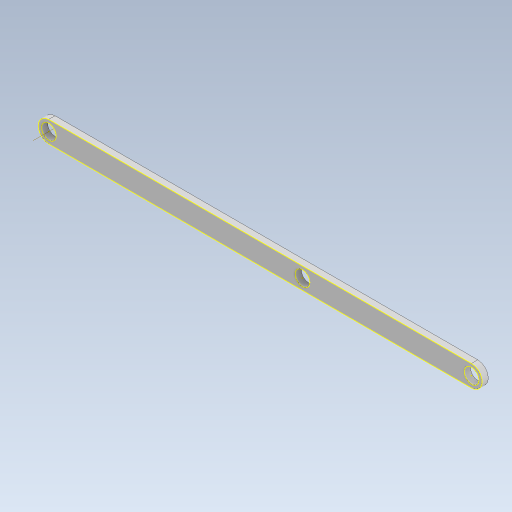
# Autodesk Inventor part: 0605_2
Saved by Autodesk Inventor 2023 (Build 270158000, 158)
## iProperties
Created: 2023-04-16
Part Number: 0605_2
Material: 一般
Document SubType Name: Modeling
Designer: JOU
Density: 1 g/cm^3
Appearance: 預設
Author: JOU
Autodesk Inventor part; units mm, degrees
ref_plane "YZ Plane" through (0, 0, 0) normal (1, 0, 0) x (0, 1, 0)
ref_plane "XZ Plane" through (0, 0, 0) normal (0, 1, 0) x (-1, 0, 0)
ref_plane "XY Plane" through (0, 0, 0) normal (0, 0, 1) x (1, 0, 0)
sketch "草圖1" plane through (0, 0, 0) normal (0, 0, 1) x (1, 0, 0)
  line L0 (-200, 0) -> (0, 0) construction
  line L1 (-200, -5) -> (0, -5)
  line L2 (0, 5) -> (-200, 5)
  arc A0 (-200, 5) -> (-200, -5) centre (-200, 0) ccw
  arc A1 (0, -5) -> (0, 5) centre (0, 0) ccw
  circle A2 centre (-200, 0) radius 3.5
  circle A3 centre (0, 0) radius 3.5
  circle A4 centre (-80, 0) radius 3.5
  point P0 (-100, 0)
  dimension "d0" = 200
  dimension "d1" = 10
  dimension "d3" = 7
  dimension "d23" = 120
  constraints: 8 end point, 5 centre point, 4 point on circle, 4 tangent, 3 coincident, 2 equal radius, 1 horizontal, 1 midpoint, 1 parallel, 1 point on line
  measures "d0" distance of L2.start L2.end
  measures "d1" distance between parallel lines of L1 L2
  measures "d3" diameter of A3
  measures "d23" distance of A2.centre A4.centre
extrude "擠出1" add sketch "草圖1" along normal blind 3
sketch "草圖4" plane through (0, 0, 3) normal (0, 0, 1) x (1, 0, 0)
  line L0 (-202.932, -0.7895) -> (-200.36, -2.1968)
  arc A0 (-200.36, -2.1968) -> (-199.64, -2.1968) centre (-200, -1.5389) ccw
  line L1 (-199.64, -2.1968) -> (-197.068, -0.7895)
  arc A1 (-197.068, -0.7895) -> (-197.068, 0.7895) centre (-197.5, 0) ccw
  line L2 (-197.068, 0.7895) -> (-199.64, 2.1968)
  arc A2 (-199.64, 2.1968) -> (-200.36, 2.1968) centre (-200, 1.5389) ccw
  line L3 (-200.36, 2.1968) -> (-202.932, 0.7895)
  arc A3 (-202.932, 0.7895) -> (-202.932, -0.7895) centre (-202.5, 0) ccw
  circle A4 centre (-200, 0) radius 1.55
  circle A5 centre (-200, 0) radius 3.5 projected
  point P0 (0, 0)
  constraints: 8 end point, 8 point on circle, 5 centre point
extrude "擠出3" [suppressed]
sketch "草圖6" plane through (0, 0, 3) normal (0, 0, 1) x (1, 0, 0)
  arc A0 (0, -5) -> (0, 5) centre (0, 0) ccw projected
  line L0 (0, 5) -> (-200, 5) projected
  arc A1 (-200, 5) -> (-200, -5) centre (-200, 0) ccw projected
  line L1 (-200, -5) -> (0, -5) projected
  circle A2 centre (-80, 0) radius 3.5 projected
  circle A3 centre (0, 0) radius 3.5 projected
  circle A4 centre (-200, 0) radius 3.5 projected
